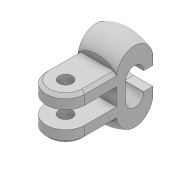
# Autodesk Inventor part: Clevis-Socket
Saved by Autodesk Inventor 2018 (Build 220112000, 112)
## iProperties
Created: 2021-04-28
Part Number: Clevis-Socket
Material: Generic
Document SubType Name: Modeling
Designer: l01767
Density: 1 g/cm^3
Appearance: Default
Author: l01767
Autodesk Inventor part; units mm, degrees
ref_plane "YZ Plane" through (0, 0, 0) normal (1, 0, 0) x (0, 1, 0)
ref_plane "XZ Plane" through (0, 0, 0) normal (0, 1, 0) x (-1, 0, 0)
ref_plane "XY Plane" through (0, 0, 0) normal (0, 0, 1) x (1, 0, 0)
sketch "Sketch1" plane through (0, 0, 0) normal (0, 0, 1) x (1, 0, 0)
  circle A0 centre (0, 0) radius 11.11
  arc A1 (-31.75, 0) -> (31.75, 0) centre (0, 0) ccw
  line L0 (31.75, 0) -> (31.75, 52.4)
  line L1 (-31.75, 0) -> (-31.75, 52.4)
  line L2 (-31.75, 74.62) -> (31.75, 74.62) construction
  line L3 (-31.75, 112.4) -> (31.75, 112.4)
  line L4 (31.75, 52.4) -> (31.75, 112.4)
  line L5 (-31.75, 112.4) -> (-31.75, 52.4)
  point P0 (0, 74.62)
  dimension "d0" = 22.22
  dimension "d3" = 31.75
  dimension "d4" = 52.4
  dimension "d7" = 74.62
  dimension "d17" = 60
  constraints: 14 end point, 4 vertical, 2 centre point, 2 coincident, 2 horizontal, 2 point on circle, 2 tangent, 2 vertical alignment, 1 horizontal alignment, 1 midpoint, 1 parallel
  measures "d0" diameter of A0
  measures "d3" radius of A1
  measures "d4" distance of L0.start L0.end
  measures "d7" distance from line of point (0, 0) L2
  measures "d17" distance of L3.start L1.end
extrude "Extrusion1" add sketch "Sketch1" along normal mid plane 70
sketch "Sketch2" plane through (0, 0, 0) normal (1, 0, 0) x (0, 1, 0)
  line L0 (52.4, 14.3) -> (-52.4, 14.3)
  line L1 (-52.4, 14.3) -> (-52.4, -14.3)
  line L2 (-52.4, -14.3) -> (52.4, -14.3)
  line L3 (52.4, -14.3) -> (52.4, 14.3)
  line L4 (52.4, 14.3) -> (-52.4, -14.3) construction
  line L5 (-52.4, 14.3) -> (52.4, -14.3) construction
  point P0 (0, 0)
  dimension "d13" = 28.6
  dimension "d14" = 52.4
  constraints: 12 end point, 2 midpoint, 2 parallel, 1 horizontal, 1 perpendicular
  measures "d13" distance of L0.end L1.end
  measures "d14" distance from line of point (0, 0) L3
extrude "Extrusion2" cut sketch "Sketch2" along normal through all both and the other way through all
sketch "Sketch3" plane through (0, 0, 0) normal (1, 0, 0) x (0, 1, 0)
  line L0 (52.4, 14.3) -> (52.4, -14.3) projected
  line L1 (112.4, -35) -> (112.4, 35) projected
  line L2 (52.4, 14.3) -> (52.4, 35)
  line L3 (52.4, -14.3) -> (52.4, -35)
  line L4 (52.4, 0) -> (112.4, 0)
  line L5 (112.4, -35) -> (112.4, -45)
  line L6 (52.4, -35) -> (52.4, -45)
  line L7 (52.4, 35) -> (52.4, 45)
  line L8 (112.4, 35) -> (112.4, 45)
  arc A0 (52.4, -45) -> (112.4, -45) centre (82.4, -35) ccw
  line L9 (112.4, -35) -> (0, -35) projected
  arc A1 (112.4, 45) -> (52.4, 45) centre (82.4, 35) ccw
  point P0 (0, 0)
  dimension "d22" = 10
  constraints: 14 end point, 6 vertical, 4 point on circle, 3 equal length, 2 centre point, 2 midpoint, 2 point on line, 1 horizontal alignment, 1 other
  measures "d22" distance of L1.start L5.end
sketch "Sketch4" plane through (-31.75, 112.4, 35) normal (0, 1, 0) x (1, 0, 0)
  line L0 (0, 70) -> (0, 0) projected
  line L1 (63.5, 0) -> (0, 0) projected
  line L2 (63.5, 70) -> (63.5, 0) projected
  line L3 (0, 70) -> (63.5, 70) projected
  line L4 (15, 15) -> (15, 55)
  line L5 (15, 55) -> (48.5, 55)
  line L6 (48.5, 55) -> (48.5, 15)
  line L7 (48.5, 15) -> (15, 15)
  point P0 (31.75, 35)
  dimension "d19" = 15
  constraints: 8 end point, 3 other
  measures "d19" distance between parallel lines of L0 L4
extrude "Extrusion3" cut sketch "Sketch4" against normal up to surface (60 mm away)
revolve "Revolution1" add sketch "Sketch3" angle 360 about axis through (0, 52.4, 0) along (0, 1, 0) contours L2 L7 A1 L8 L1 L4 L0
chamfer "Chamfer1" distance 5 angle 45 6 edges at (31.75, 26.2, 35) (0, -31.75, 35) (-31.75, 26.2, 35) (31.75, 26.2, -35) (0, -31.75, -35) (-31.75, 26.2, -35)
sketch "Sketch5" plane through (0, 0, 0) normal (0, 0, 1) x (1, 0, 0)
  line L0 (31.75, 52.4) -> (31.75, 0) projected
  line L1 (31.75, 52.4) -> (91.75, 52.4)
  line L2 (91.75, 52.4) -> (91.75, 112.4)
  line L3 (91.75, 112.4) -> (31.75, 112.4)
  line L4 (31.75, 112.4) -> (31.75, 52.4)
  line L5 (45, 112.4) -> (-45, 112.4) construction
  line L6 (0, 52.4) -> (0, 112.4)
  line L7 (-31.75, 52.4) -> (-31.75, 0)
  line L8 (-31.75, 52.4) -> (-91.75, 52.4)
  line L9 (-91.75, 52.4) -> (-91.75, 112.4)
  line L10 (-91.75, 112.4) -> (-31.75, 112.4)
  line L11 (-31.75, 112.4) -> (-31.75, 52.4)
  line L12 (-45, 112.4) -> (45, 112.4) construction
  point P0 (0, 0)
  dimension "d28" = 60
  constraints: 22 end point, 7 symmetric about line, 2 parallel, 1 collinear, 1 horizontal, 1 midpoint, 1 perpendicular
  measures "d28" distance of L0.start L1.end
extrude "Extrusion4" cut sketch "Sketch5" along normal through all both and the other way through all
sketch "Sketch6" plane through (0, 0, 0) normal (1, 0, 0) x (0, 1, 0)
  line L0 (112.4, 31.8895) -> (112.4, -31.8895) projected
  line L1 (112.4, 0) -> (112.4, 15)
  line L2 (112.4, 15) -> (97.4, 15)
  arc A0 (97.4, 15) -> (67.4, 15) centre (82.4, 15) ccw
  line L3 (112.4, 0) -> (67.4, 0)
  line L4 (67.4, 0) -> (67.4, 15)
  point P0 (0, 0)
  dimension "d31" = 15
  dimension "d32" = 15
  dimension "d34" = 15
  constraints: 8 end point, 3 point on line, 2 point on circle, 1 centre point, 1 horizontal, 1 midpoint, 1 perpendicular, 1 vertical
  measures "d31" distance of L1.start L1.end
  measures "d32" distance of L1.end L2.end
  measures "d34" radius of A0
revolve "Revolution2" cut sketch "Sketch6" angle 360 about axis through (0, 112.4, 0) along (0, -1, 0)
sketch "Sketch7" plane through (31.75, 0, 14.3) normal (1, 0, 0) x (0, 0, -1)
  line L0 (29.3, 67.4) -> (-0.7, 67.4) projected
  line L1 (29.3, 97.4) -> (-0.7, 97.4) construction
  arc A0 (-0.7, 97.4) -> (-0.7, 67.4) centre (-0.7, 82.4) ccw
  arc A1 (29.3, 67.4) -> (29.3, 97.4) centre (29.3, 82.4) ccw
  line L2 (46.1895, 112.4) -> (-17.5895, 112.4) construction
  line L3 (29.3, 112.4) -> (29.3, 97.4)
  line L4 (29.3, 112.4) -> (-0.7, 112.4)
  line L5 (-0.7, 97.4) -> (-0.7, 112.4)
  point P0 (14.3, 0)
  constraints: 6 end point, 4 point on circle, 2 centre point, 2 point on line, 2 tangent, 2 vertical
extrude "Extrusion5" cut sketch "Sketch7" against normal up to surface (31.75 mm away)
body "Solid1"
